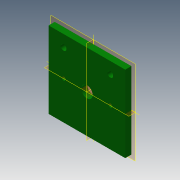
# Autodesk Inventor part: HbBatteryPcb02
Saved by Autodesk Inventor 2015 SP1 (Build 190203100, 203)
## iProperties
Created: 2015-12-21
Part Number: HbBatteryPcb02
Material: ABS プラスチック
Document SubType Name: Modeling
Designer: Yamaura
Density: 1.06 g/cm^3
Appearance: 濃い緑
Author: Yamaura
Autodesk Inventor part; units mm, degrees
sketch "スケッチ1" plane through (0, 0, 0) normal (0, 0, 1) x (1, 0, 0)
  line L0 (-10, -10) -> (10, -10)
  line L1 (10, -10) -> (10, 10)
  line L2 (10, 10) -> (-10, 10)
  line L3 (-10, 10) -> (-10, -10)
  line L4 (-10, -10) -> (10, 10) construction
  line L5 (10, -10) -> (-10, 10) construction
  point P0 (0, 0)
  dimension "d0" = 20
  dimension "d1" = 20
  constraints: 12 end point, 2 midpoint, 2 parallel, 1 horizontal, 1 perpendicular
  measures "d0" distance of L2.end L1.end
  measures "d1" distance of L1.end L0.end
extrude "押し出し1" add sketch "スケッチ1" along normal blind 1.6
sketch "スケッチ2" plane through (0, 0, 0) normal (0, 0, 1) x (1, 0, 0)
  circle A0 centre (-6.1, 7) radius 0.75
  circle A1 centre (6.1, 7) radius 0.75
  point P0 (0, 0)
  dimension "d9" = 1.5
  dimension "d10" = 7
  dimension "d11" = 6.1
  dimension "d14" = 1.5
  dimension "d15" = 12.2
  constraints: 2 centre point
  measures "d9" diameter of A0
  measures "d10" vertical distance of A0.centre point (0, 0)
  measures "d11" horizontal distance of A0.centre point (0, 0)
  measures "d14" diameter of A1
  measures "d15" distance of A1.centre A0.centre
extrude "押し出し2" cut sketch "スケッチ2" along normal blind 1.6
sketch "スケッチ3" plane through (0, 0, 0) normal (0, 0, 1) x (1, 0, 0)
  circle A0 centre (-6.1, 0) radius 0.5
  circle A1 centre (6.1, 0) radius 0.5
  point P0 (0, 0)
  dimension "d16" = 1
  dimension "d17" = 6.1
  dimension "d18" = 1
  dimension "d19" = 6.1
  constraints: 2 centre point
  measures "d16" diameter of A0
  measures "d17" distance of A0.centre point (0, 0)
  measures "d18" diameter of A1
  measures "d19" distance of point (0, 0) A1.centre
extrude "押し出し3" cut sketch "スケッチ3" along normal blind 1.6
sketch "スケッチ4" plane through (0, 0, 0) normal (0, 0, 1) x (1, 0, 0)
  circle A0 centre (0, 0) radius 1.5
  dimension "d22" = 3
  constraints: 1 centre point, 1 coincident
  measures "d22" diameter of A0
extrude "押し出し4" cut sketch "スケッチ4" along normal blind 3
equation "\"d23\" = d22"
